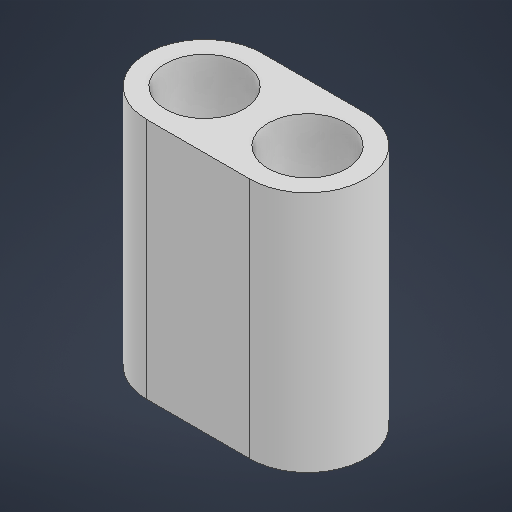
# Autodesk Inventor part: BackpackFrameLinearJoint
Saved by Autodesk Inventor 2026.1 (Build 301233020, 233B)
## iProperties
Created: 2025-10-30
Part Number: BackpackFrameLinearJoint
Material: Generic
Document SubType Name: Modeling
Designer: skybound
Density: 1 g/cm^3
Appearance: Default
Author: skybound
Autodesk Inventor part; units mm, degrees
ref_plane "YZ Plane" through (0, 0, 0) normal (1, 0, 0) x (0, 1, 0)
ref_plane "XZ Plane" through (0, 0, 0) normal (0, 1, 0) x (-1, 0, 0)
ref_plane "XY Plane" through (0, 0, 0) normal (0, 0, 1) x (1, 0, 0)
sketch "Sketch1" plane through (0, 0, 0) normal (0, 1, 0) x (-1, 0, 0)
  circle A0 centre (4.25, 0) radius 3.25
  circle A1 centre (-4.25, 0) radius 3.25
  line L0 (4.25, 0) -> (-4.25, 0) construction
  line L1 (0, 0) -> (0, -13.2538) construction
  circle A2 centre (4.25, 0) radius 4.75
  circle A3 centre (-4.25, 0) radius 4.75
  line L2 (4.25, -4.75) -> (-4.25, -4.75)
  line L3 (4.25, 4.75) -> (-4.25, 4.75)
  dimension "d0" = 6.5
  dimension "d1" = 8.5
  dimension "d2" = 1.5
  dimension "d3" = 1.5
  constraints: 8 end point, 4 centre point, 4 point on circle, 4 tangent, 1 equal radius, 1 horizontal, 1 midpoint, 1 vertical, 1 other
  measures "d0" diameter of A1
  measures "d1" distance of L0.start L0.end
  measures "d2" radial gap between concentric circles of A0 A2
  measures "d3" radial gap between concentric circles of A1 A3
extrude "Extrusion1" add sketch "Sketch1" along normal blind 20
body "Solid1"
